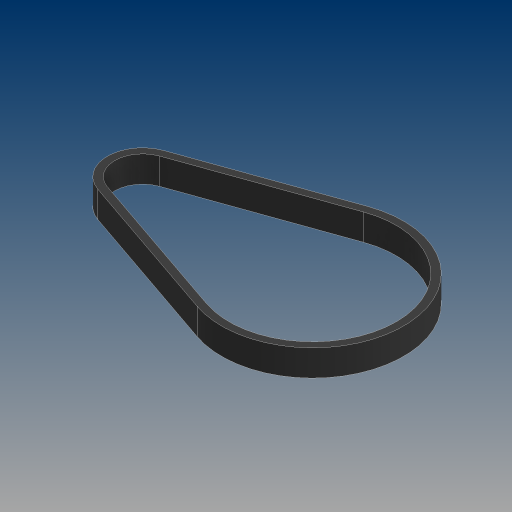
# Autodesk Inventor part: INTK_009_Belt1
Saved by Autodesk Inventor 2024.3 (Build 283343000, 343)
## iProperties
Created: 2024-08-07
Part Number: INTK_009_Belt1
Material: Rubber, Silicone
Document SubType Name: Modeling
Designer: Kenji
Density: 1.25 g/cm^3
Appearance: Rubber - Black
Author: Kenji
Autodesk Inventor part; units mm, degrees
ref_plane "YZ Plane" through (0, 0, 0) normal (1, 0, 0) x (0, 1, 0)
ref_plane "XZ Plane" through (0, 0, 0) normal (0, 1, 0) x (-1, 0, 0)
ref_plane "XY Plane" through (0, 0, 0) normal (0, 0, 1) x (1, 0, 0)
sketch "Sketch1" plane through (0, 0, 0) normal (0, 1, 0) x (-1, 0, 0)
  circle A0 centre (0, 0) radius 28.6512 construction
  line L0 (0, 0) -> (0, 28.6512) construction
  line L1 (0, 0) -> (57.9379, 0.3498) construction
  circle A1 centre (57.9379, 0.3498) radius 9.5504 construction
  line L2 (61.0319, 9.3851) -> (9.282, 27.106)
  line L3 (61.1408, -8.6475) -> (9.6086, -26.992)
  arc A2 (61.1408, -8.6475) -> (61.0319, 9.3851) centre (57.9379, 0.3498) ccw
  arc A3 (9.282, 27.106) -> (9.6086, -26.992) centre (0, 0) ccw
  line L4 (10.4604, -29.3849) -> (61.9926, -11.0404)
  arc A4 (61.9926, -11.0404) -> (61.8548, 11.7881) centre (57.9379, 0.3498) ccw
  line L5 (61.8548, 11.7881) -> (10.1049, 29.509)
  arc A5 (10.1049, 29.509) -> (10.4604, -29.3849) centre (0, 0) ccw
  dimension "d0" = 57.3024
  dimension "d1" = 57.939
  dimension "d2" = 89.654
  dimension "d3" = 19.1008
  dimension "d4" = 2.54
  constraints: 13 point on circle, 12 end point, 8 tangent, 6 centre point, 2 coincident, 1 vertical, 3 other
  measures "d0" diameter of A0
  measures "d1" distance of L0.start L1.end
  measures "d2" angle of L0 L1
  measures "d3" diameter of A1
  measures "d4" distance between parallel lines of L3 L4
extrude "Extrusion1" add sketch "Sketch1" along normal blind 8.9916
body "Solid1"
